Autodesk Fusion 360 part; units mm, degrees
note: some values were not read from the file. Chosen so that the rebuilt part matches the saved one: which face or edge a step refers to. Set by a fixed rule: which sketch regions a step uses.
(part 4 of 4)
sketch "Sketch11 (2)" plane through (0, 0, 0) normal (0, 1, 0) x (1, 0, 0) in component "Lid"
  line L0 (-117.5, -16.1) -> (49.7, -16.1)
  line L1 (49.7, -16.1) -> (49.7, 22.1)
  line L2 (49.7, 22.1) -> (-117.5, 22.1)
  line L3 (-117.5, 22.1) -> (-117.5, -16.1)
  line L4 (59.75, -26) -> (-127.75, -26)
  line L5 (-127.75, -26) -> (-127.75, 32)
  line L6 (-115.5, -14.1) -> (47.7, -14.1)
  line L7 (47.7, -14.1) -> (47.7, 20.1)
  line L8 (47.7, 20.1) -> (-115.5, 20.1)
  line L9 (-115.5, 20.1) -> (-115.5, -14.1)
  line L10 (-76.2, -14.1) -> (-74.2, -14.1)
  line L11 (-74.2, -14.1) -> (-74.2, 20.1)
  line L12 (-74.2, 20.1) -> (-76.2, 20.1)
  line L13 (-76.2, 20.1) -> (-76.2, -14.1)
  line L14 (-32.9, 20.1) -> (-34.9, 20.1)
  line L15 (-34.9, 20.1) -> (-34.9, -14.1)
  line L16 (-34.9, -14.1) -> (-32.9, -14.1)
  line L17 (-32.9, -14.1) -> (-32.9, 20.1)
  line L18 (8.4, 20.1) -> (6.4, 20.1)
  line L19 (6.4, 20.1) -> (6.4, -14.1)
  line L20 (6.4, -14.1) -> (8.4, -14.1)
  line L21 (8.4, -14.1) -> (8.4, 20.1)
  line L22 (59.75, 32) -> (59.75, -26)
  dimension "d1645" = 38.2
  dimension "d1646" = 9.9
  dimension "d1647" = 10.25
  dimension "d1648" = 34.2
  dimension "d1649" = 2
  dimension "d1650" = 2
  dimension "d1651" = 2
  dimension "d1652" = 2
  dimension "d1653" = 39.3
  dimension "d1654" = 2
  dimension "d1655" = 39.3
  dimension "d1656" = 2
  dimension "d1657" = 39.3
  dimension "d1661" = 39.3
  constraint horizontal L0
  constraint vertical L1
  constraint horizontal L2
  constraint vertical L3
  constraint horizontal L6
  constraint vertical L7
  constraint horizontal L8
  constraint vertical L9
  constraint horizontal L10
  constraint vertical L11
  constraint horizontal L12
  constraint vertical L13
  constraint coincident L8 L11.end
  constraint coincident L6 L10.start
  constraint horizontal L14
  constraint vertical L15
  constraint horizontal L16
  constraint vertical L17
  constraint coincident L8 L14.start
  constraint horizontal L18
  constraint vertical L19
  constraint horizontal L20
  constraint vertical L21
  constraint coincident L8 L18.start
  measures "d1645" distance of L0.start L2.end
  measures "d1646" distance of L0 L4
  measures "d1647" distance of L3 L5
  measures "d1648" distance of L6.start L8.end
  measures "d1649" distance of L0 L6
  measures "d1650" distance of L1 L7
  measures "d1651" distance of L3 L9
  measures "d1652" distance of L11 L13
  measures "d1653" distance of L9 L13
  measures "d1654" distance of L14.start L14.end
  measures "d1655" distance of L11 L15
  measures "d1656" distance of L18.start L18.end
  measures "d1657" distance of L17 L19
  measures "d1661" distance of L7 L21
extrude "Extrude10''" [suppressed] in component "Lid"
sketch "Sketch13 (3)" plane through (0, 38.25, 0) normal (0, 1, 0) x (-1, 0, 0) in component "Lid"
  circle A0 centre (54.55, -2) radius 14.6
  circle A1 centre (13.35, -2) radius 14.6
  circle A2 centre (95.75, -2) radius 14.6
  circle A3 centre (-27.85, -2) radius 14.6
  line L0 (-59.75, -32) -> (127.75, -32)
  line L1 (127.75, -32) -> (127.75, 26)
  line L2 (-59.75, 26) -> (-59.75, -32)
  circle A4 centre (122.75, -27.8) radius 2
  circle A5 centre (122.75, 21.8) radius 2
  circle A6 centre (-54.75, -27.8) radius 2
  circle A7 centre (-54.75, 21.8) radius 2
  circle A8 centre (122.75, 21.8) radius 2
  circle A9 centre (-54.75, -27.8) radius 2
  circle A10 centre (122.75, -27.8) radius 2
  circle A11 centre (-54.75, 21.8) radius 2
  line L3 (127.75, 26) -> (-59.75, 26)
  dimension "d1666" = 4
  dimension "d1667" = 4
  dimension "d1668" = 4
  dimension "d1669" = 4
  measures "d1666" diameter of A5
  measures "d1667" diameter of A4
  measures "d1668" diameter of A7
  measures "d1669" diameter of A6
extrude "Extrude11''" [suppressed] in component "Lid"
sketch "Sketch13 (4)" plane through (0, 6, 0) normal (0, 1, 0) x (-1, 0, 0) in component "Box"
  circle A0 centre (84.75, -30) radius 1.0877
sketch "Sketch20" plane through (0, 3, 0) normal (0, 1, 0) x (-1, 0, 0) in component "Button Base"
component "Box" placed x (1, 0, 0) y (0, 1, 0) z (0, 0, 1) at (-103.0128, 41.0959, 7.7419)
component "Lid" placed x (1, 0, 0) y (0, 1, 0) z (0, 0, 1) at (-74.0128, 41.0959, -34.2581)
component "Button" placed x (-1, 0, 0) y (0, 1, 0) z (0, 0, -1) at (-147.5499, 44.4152, 72.8738)
component "Button Base" placed x (-1, 0, 0) y (0, 1, 0) z (0, 0, -1) at (-103.2628, 54.0959, 7.4419)
equation "capL = 22.5 mm"
equation "baseWidth = 37 mm"
equation "baseHeight = 5 mm"
equation "capsenseWidth = 17.4 mm"
equation "capsenseLength = 22.4 mm"
equation "capsenseBase_length = capsenseLength + 3 mm"
equation "capsenseBase_width = 34 mm"
equation "screwHoleID = 4 mm"
equation "screwHole_OD = 6.1 mm"
equation "acrlyic_coverOD = 28 mm"
equation "acrlyicThick = 3.175 mm"
equation "capsenseBase_height = 3 mm"
equation "capsenseThick = 1.5 mm"
equation "coverH = 11 mm"
equation "acrylicCoverOD = 28 mm"
equation "magnL = 5.5 mm"
equation "toleranceFit = 0.2 mm"
equation "magOD = 5.9 mm" comment "5.88 mm"
equation "buttonOD = 28 mm"
equation "buttonH = 11 mm"
equation "baseMagW = 48 mm"
equation "coverMagH = 15 mm"
equation "screwHoleDFC = 21 mm"
equation "d178 = 28.40 mm"
equation "NeopixelCoverSupportOD = 26.4 mm"
equation "screwHeadheight = 1.2954 mm"
equation "baseLipH = 3.175 mm"
equation "capBaseW = 39 mm"
equation "capBaseL = 39 mm"
equation "magnetDepth = -2.4 mm" comment "1.43 mm"
equation "magCentertoCapsense = 4.2 mm"
equation "boxW = 70 mm"
equation "boxH = 33 mm"
equation "boxTopH = 3 mm"
equation "boxL = 100 mm"
equation "d1 = 17 mm"
equation "d2 = 7.5 mm"
equation "d3 = 8 mm"
equation "d5 = 3.175 mm"
equation "d12 = 135 deg"
equation "d13 = 4 mm"
equation "d7 = 30 mm"
equation "d8 = 0.0 deg"
equation "d9 = 30 mm"
equation "d10 = 0.0 deg"
equation "d43 = capsenseWidth"
equation "d44 = capsenseLength"
equation "d45 = ( 34 / 2 ) * 1 mm"
equation "d46 = capsenseWidth / 2"
equation "d47 = 9 mm"
equation "d48 = -10.00 mm"
equation "d49 = 0.0 deg"
equation "d50 = magOD"
equation "d52 = 17 mm"
equation "d54 = 4.2 mm"
equation "d55 = 4.2 mm"
equation "d56 = 4.2 mm"
equation "d57 = 4.2 mm"
equation "d58 = capsenseLength / 2"
equation "d59 = capsenseWidth / 2"
equation "d61 = magnetDepth"
equation "d62 = 0.0 deg"
equation "d63 = 10.00 mm"
equation "d64 = capsenseThick + 0.2 mm"
equation "d67 = capsenseWidth"
equation "d69 = ( 34 / 2 ) * 1 mm"
equation "d70 = capsenseWidth / 2"
equation "d72 = 45 deg"
equation "d73 = 2.268 mm"
equation "d74 = 2.268048 mm"
equation "d75 = 135 deg"
equation "d65 = 10.00 mm"
equation "d66 = 0.0 deg"
equation "d76 = 39.00 mm"
equation "d77 = 0.0 deg"
equation "d78 = 1"
equation "d79 = 2"
equation "d80 = 0 mm"
equation "d81 = 39.00 mm"
equation "d82 = -20.00 mm"
equation "d83 = 0.0 deg"
equation "d106 = magnetDepth"
equation "d107 = 0.0 deg"
equation "d116 = screwHoleID"
equation "d117 = 5 mm"
equation "d118 = 5 mm"
equation "d119 = 4 mm"
equation "d120 = 4 mm"
equation "d121 = -4.00 mm"
equation "d122 = 0.0 deg"
equation "d123 = screwHole_OD"
equation "d125 = -screwHeadheight"
equation "d126 = 0.0 deg"
equation "d127 = 2"
equation "d128 = 1"
equation "d129 = 69.00 mm"
equation "d130 = 0.00 mm"
equation "d132 = 10.00 mm"
equation "d133 = 10 mm"
equation "d136 = 8.00 mm"
equation "d137 = 8 mm"
equation "d138 = 10 mm"
equation "d139 = 10 mm"
equation "d134 = -4.00 mm"
equation "d135 = 0.0 deg"
equation "d229 = 3.175 mm"
equation "d230 = 4.825 mm"
equation "d388 = 2 mm"
equation "d389 = 2 mm"
equation "d86 = capBaseW"
equation "d87 = capBaseL"
equation "d88 = 3 mm"
equation "d89 = 0.0 deg"
equation "d90 = buttonOD"
equation "d114 = capBaseW / 2"
equation "d115 = capBaseW / 2"
equation "d91 = buttonH + 3 mm"
equation "d92 = 0.0 deg"
equation "d365 = ( 39 / 2 ) * 1 mm"
equation "d367 = ( 39 / 2 ) * 1 mm"
equation "d368 = capsenseWidth"
equation "d369 = capsenseLength"
equation "d370 = capsenseLength / 2"
equation "d371 = capsenseWidth / 2"
equation "d372 = magOD"
equation "d373 = 4.2 mm"
equation "d374 = 4.2 mm"
equation "d375 = 4.2 mm"
equation "d376 = 4.2 mm"
equation "d108 = magnetDepth"
equation "d109 = 0.0 deg"
equation "d110 = 2 mm"
equation "d377 = 2 mm"
equation "d112 = 7 mm"
equation "d113 = 0.0 deg"
equation "d140 = buttonOD + 1 mm"
equation "d145 = 3 mm"
equation "d146 = 0.0 deg"
equation "d147 = 1 mm"
equation "d148 = 1 mm"
equation "d149 = boxW"
equation "d150 = 60 mm"
equation "d151 = 50 mm"
equation "d152 = 0.0 deg"
equation "d153 = 50 mm"
equation "d154 = 0 deg"
equation "d155 = 20 mm"
equation "d156 = 20 mm"
equation "d157 = 10 mm"
equation "d158 = 10 mm"
equation "d167 = 3 mm"
equation "d170 = 3 mm"
equation "d171 = 3 mm"
equation "d260 = 3 mm"
equation "d172 = -23.00 mm"
equation "d173 = 0.0 deg"
equation "d193 = 70 mm"
equation "d194 = 49.999997 mm"
equation "d195 = 35 mm"
equation "d196 = screwHoleID"
equation "d197 = screwHoleID"
equation "d198 = 5 mm"
equation "d199 = 5 mm"
equation "d215 = 50 mm"
equation "d216 = boxW / 2"
equation "d217 = 25 mm"
equation "d218 = 70 mm"
equation "d219 = 35 mm"
equation "d220 = 8 mm"
equation "d221 = 8 mm"
equation "d222 = 4 mm"
equation "d223 = 5.000003 mm"
equation "d224 = 5.00 mm"
equation "d225 = 4 mm"
equation "d226 = 4 mm"
equation "d228 = 4 mm"
equation "d202 = -10 mm"
equation "d203 = 0.0 deg"
equation "d231 = -20.00 mm"
equation "d232 = 60 mm"
equation "d233 = 3 mm"
equation "d234 = 25.00 mm"
equation "d235 = 5 mm"
equation "d236 = -5.00 mm"
equation "d237 = 0.0 deg"
equation "d238 = 95.00 mm"
equation "d239 = 0.0 deg"
equation "d263 = 2 mm"
equation "d264 = 2 mm"
equation "d265 = 2 mm"
equation "d337 = 2 mm"
equation "d266 = -2 mm"
equation "d267 = -3 mm"
equation "d268 = 0.0 deg"
equation "d274 = 2 mm"
equation "d275 = 2 mm"
equation "d276 = 2 mm"
equation "d280 = 2 mm"
equation "d277 = -2 mm"
equation "d278 = -3 mm"
equation "d279 = 0.0 deg"
equation "d281 = 2 mm"
equation "d282 = 2 mm"
equation "d283 = 2 mm"
equation "d284 = 2 mm"
equation "d285 = 3 mm"
equation "d286 = 5 mm"
equation "d287 = 3 mm"
equation "d288 = -5.00 mm"
equation "d289 = 0.0 deg"
equation "d290 = 2 mm"
equation "d293 = 5 mm"
equation "d294 = 2 mm"
equation "d295 = -2.00 mm"
equation "d296 = 0.0 deg"
equation "d344 = 2 mm"
equation "d345 = 2 mm"
equation "d346 = -1.00 mm"
equation "d347 = 0.0 deg"
equation "d348 = 2 mm"
equation "d349 = 2 mm"
equation "d350 = -2 mm"
equation "d351 = 0.0 deg"
equation "d378 = -50.00 mm"
equation "d379 = 0.0 deg"
equation "d380 = 2 mm"
equation "d381 = 2 mm"
equation "d382 = -1 mm"
equation "d383 = -3.00 mm"
equation "d384 = 0.0 deg"
equation "d390 = -2 mm"
equation "d391 = -2 deg"
equation "d240 = 70 mm"
equation "d241 = 100 mm"
equation "d245 = 3.175 mm"
equation "d246 = 0.0 deg"
equation "d247 = 39 mm"
equation "d248 = 79 mm"
equation "d249 = ( 65.8 / 2 ) * 1 mm"
equation "d250 = ( 95.8 / 2 ) * 1 mm"
equation "d251 = 39 mm"
equation "d253 = buttonOD + 1 mm"
equation "d254 = ( 39 / 2 ) * 1 mm"
equation "d255 = 39 mm"
equation "d256 = ( 39 / 2 ) * 1 mm"
equation "d257 = ( 39 / 2 ) * 1 mm"
equation "d258 = -20.00 mm"
equation "d259 = 0.0 deg"
equation "d308 = 3.5 mm"
equation "d311 = 3 mm"
equation "d312 = 3.5 mm"
equation "d320 = 3 mm"
equation "d338 = 9 mm"
equation "d385 = 58.80 mm"
equation "d386 = 55.80 mm"
equation "d387 = 9 mm"
equation "d315 = -4 mm"
equation "d316 = 0.0 deg"
equation "d321 = 2.5 mm"
equation "d322 = 1.5 mm"
equation "d323 = 3 mm"
equation "d324 = 3 mm"
equation "d325 = 1.5 mm"
equation "d326 = 0.0 deg"
equation "d327 = 2.5 mm"
equation "d328 = 3 mm"
equation "d330 = 1.5 mm"
equation "d331 = 0.0 deg"
equation "d332 = 2.5 mm"
equation "d333 = 3 mm"
equation "d334 = 3 mm"
equation "d335 = 1.5 mm"
equation "d336 = 0.0 deg"
equation "d352 = 95.5 mm"
equation "d353 = 55 mm - 3.175 mm - 0.2 mm + 3 mm"
equation "d354 = 1.6 mm"
equation "d355 = 0.0 deg"
equation "d356 = 35 mm"
equation "d357 = 45 deg"
equation "d358 = 135 deg"
equation "d359 = ( 95.5 / 2 ) * 1 mm"
equation "d360 = ( 35 / 2 ) * 1 mm"
equation "d361 = -10.00 mm"
equation "d362 = 0.0 deg"
equation "d405 = boxH"
equation "d407 = Button4BaseL + 6 mm + 0.5 mm"
equation "d408 = 52 mm + 6 mm"
equation "d431 = screwHoleID"
equation "d460 = capsenseLength"
equation "d461 = capsenseWidth"
equation "d462 = capsenseWidth / 2"
equation "d468 = capsenseLength / 2"
equation "d500 = 3.3 mm - 0.8 mm"
equation "d503 = capsenseWidth / 2"
equation "d506 = magOD"
equation "d507 = magCentertoCapsense"
equation "d509 = magCentertoCapsense"
equation "d510 = magCentertoCapsense"
equation "d511 = magnetDepth"
equation "d517 = capsenseLength / 2"
equation "d541 = capsenseLength / 2"
equation "d542 = capsenseWidth / 2"
equation "d552 = 13 mm - 5 mm"
equation "d570 = screwHoleID"
equation "d586 = screwHoleID"
equation "d612 = magnetDepth"
equation "d614 = 3 mm - magnetDepth"
equation "d616 = buttonOD"
equation "d617 = ( 34.2 / 2 ) * 1 mm"
equation "d620 = ( 39.2 / 2 ) * 1 mm"
equation "d621 = buttonH"
equation "d624 = 39.2 mm - 0.5 mm"
equation "d625 = 34.2 mm - 0.5 mm"
equation "Button4BaseL = 167 mm"
equation "d684 = capsenseLength"
equation "d685 = capsenseWidth"
equation "d686 = ( 10.5 * 2 ) * 1 mm - 2.2 mm"
equation "d687 = capsenseLength"
equation "d688 = capsenseWidth"
equation "d690 = capsenseLength"
equation "d691 = capsenseWidth"
equation "d738 = Button4BaseL"
equation "Button4BaseWidth = 38.2 mm"
equation "d743 = magCentertoCapsense"
equation "d744 = magOD"
equation "d745 = magCentertoCapsense"
equation "d748 = capsenseLength / 2"
equation "d749 = capsenseLength / 2"
equation "d750 = magCentertoCapsense"
equation "d751 = magCentertoCapsense"
equation "d752 = capsenseWidth / 2"
equation "d755 = magCentertoCapsense"
equation "d760 = magCentertoCapsense"
equation "d761 = magOD"
equation "d765 = capsenseLength / 2"
equation "d766 = capsenseLength / 2"
equation "d767 = magCentertoCapsense"
equation "d768 = magCentertoCapsense"
equation "d769 = capsenseWidth / 2"
equation "d770 = magCentertoCapsense"
equation "d771 = magOD"
equation "d774 = capsenseLength / 2"
equation "d775 = capsenseLength / 2"
equation "d777 = magCentertoCapsense"
equation "d780 = magCentertoCapsense"
equation "d784 = magCentertoCapsense"
equation "d791 = screwHole_OD"
equation "d792 = screwHole_OD"
equation "d796 = -screwHeadheight"
equation "d798 = screwHoleID"
equation "d799 = screwHoleID"
equation "d803 = screwHoleID"
equation "d850 = buttonBaseW"
equation "buttonBaseL = 37.5 mm"
equation "buttonBaseW = 33.5 mm"
equation "d853 = magnetDepth"
equation "d860 = 3 mm + magnetDepth"
equation "d862 = ( 38 / 2 ) * 1 mm"
equation "d863 = ( 33.5 / 2 ) * 1 mm"
equation "d864 = buttonOD"
equation "d867 = buttonH"
equation "d869 = Button4BaseWidth"
equation "d870 = Button4BaseL"
equation "d877 = screwHoleID"
equation "d897 = screwHoleID"
equation "d1030 = screwHoleID"
equation "d1060 = ( 187.5 / 2 ) * 1 mm"
equation "d1315 = boxH - 18 mm - 3 mm"
equation "d1323 = ( 43.3 / 2 ) * 1 mm"
equation "d1328 = ( 43.3 / 2 ) * 1 mm + 0.5 mm"
equation "d1346 = 43 mm + 8 mm"
equation "d1475 = buttonOD"
equation "d1477 = ( 33.5 / 2 ) * 1 mm"
equation "d1549 = ( 38 / 2 ) * 1 mm"
equation "d1550 = ( 33.5 / 2 ) * 1 mm"
equation "d1555 = ( 38 / 2 ) * 1 mm"
equation "d1557 = ( 33.5 / 2 ) * 1 mm"
equation "buttonOD_1 = 28 mm"
equation "d612_1 = magnetDepth_1"
equation "d614_1 = 3 mm - magnetDepth_1"
equation "d616_1 = buttonOD_2"
equation "d617_1 = ( 34.2 / 2 ) * 1 mm"
equation "d620_1 = ( 39.2 / 2 ) * 1 mm"
equation "d621_1 = buttonH_1"
equation "d624_1 = 39.2 mm - 0.5 mm"
equation "d625_1 = 34.2 mm - 0.5 mm"
equation "d850_1 = buttonBaseW_1"
equation "d853_1 = magnetDepth_1"
equation "d860_1 = 3 mm + magnetDepth_1"
equation "d862_1 = ( 38 / 2 ) * 1 mm"
equation "d863_1 = ( 33.5 / 2 ) * 1 mm"
equation "d864_1 = buttonOD_2"
equation "buttonOD_2 = 28 mm"
equation "buttonH_1 = 15 mm"
equation "magnetDepth_1 = -1.8 mm" comment "1.43 mm"
equation "buttonBaseW_1 = 33.5 mm"
equation "d612_2 = magnetDepth_2"
equation "d614_2 = 3 mm - magnetDepth_2"
equation "d616_2 = buttonOD_3"
equation "d617_2 = ( 34.2 / 2 ) * 1 mm"
equation "d620_2 = ( 39.2 / 2 ) * 1 mm"
equation "d621_2 = buttonH_2"
equation "d624_2 = 39.2 mm - 0.5 mm"
equation "d625_2 = 34.2 mm - 0.5 mm"
equation "d850_2 = buttonBaseW_2"
equation "d853_2 = magnetDepth_2"
equation "d860_2 = 3 mm + magnetDepth_2"
equation "d862_2 = ( 38 / 2 ) * 1 mm"
equation "d863_2 = ( 33.5 / 2 ) * 1 mm"
equation "d864_2 = buttonOD_3"
equation "buttonOD_3 = 28 mm"
equation "buttonH_2 = 15 mm"
equation "magnetDepth_2 = -1.8 mm" comment "1.43 mm"
equation "buttonBaseW_2 = 33.5 mm"
equation "d612_3 = magnetDepth_3"
equation "d614_3 = 3 mm - magnetDepth_3"
equation "d616_3 = buttonOD_4"
equation "d617_3 = ( 34.2 / 2 ) * 1 mm"
equation "d620_3 = ( 39.2 / 2 ) * 1 mm"
equation "d621_3 = buttonH_3"
equation "d624_3 = 39.2 mm - 0.5 mm"
equation "d625_3 = 34.2 mm - 0.5 mm"
equation "d850_3 = buttonBaseW_3"
equation "d853_3 = magnetDepth_3"
equation "d860_3 = 3 mm + magnetDepth_3"
equation "d862_3 = ( 38 / 2 ) * 1 mm"
equation "d863_3 = ( 33.5 / 2 ) * 1 mm"
equation "d864_3 = buttonOD_4"
equation "buttonOD_4 = 28 mm"
equation "buttonH_3 = 15 mm"
equation "magnetDepth_3 = -1.8 mm" comment "1.43 mm"
equation "buttonBaseW_3 = 33.5 mm"
equation "d1596 = ( 187.5 / 2 ) * 1 mm"
equation "d1597 = ( 58 / 2 ) * 1 mm"
equation "d1665 = -screwHeadheight"
equation "d1666 = screwHoleID"
equation "d1667 = screwHoleID"
equation "d1668 = screwHoleID"
equation "d1669 = screwHoleID"
named bodies: "Test", "Button Bottom", "Button Top", "Button Cylinder"
